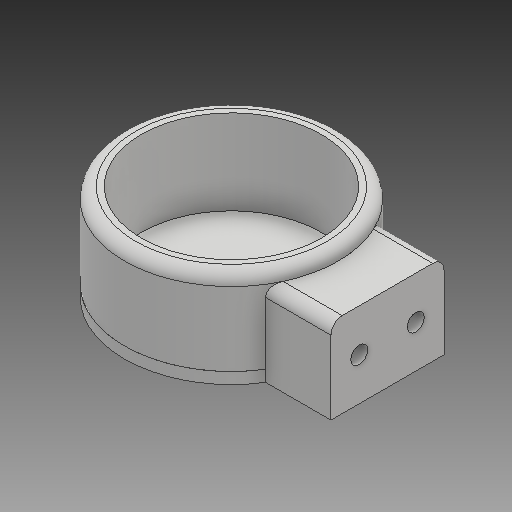
# Autodesk Inventor part: Counter_Support_Ceramic_Base
Saved by Autodesk Inventor 2017 (Build 210142000, 142)
## iProperties
Created: 2020-01-10
Part Number: Counter_Support_Ceramic_Base
Material: Generic
Document SubType Name: Modeling
Designer: Christian
Density: 1 g/cm^3
Appearance: Default
Author: Christian
Autodesk Inventor part; units mm, degrees
ref_plane "YZ Plane" through (0, 0, 0) normal (1, 0, 0) x (0, 1, 0)
ref_plane "XZ Plane" through (0, 0, 0) normal (0, 1, 0) x (-1, 0, 0)
ref_plane "XY Plane" through (0, 0, 0) normal (0, 0, 1) x (1, 0, 0)
sketch "Tube_Base_Skt" plane through (0, 0, 0) normal (0, 0, 1) x (1, 0, 0)
  circle A0 centre (0, 0) radius 18.9
  dimension "d5" = 37.8
  constraints: 1 centre point, 1 coincident
  measures "d5" diameter of A0
extrude "Tube_Base" add sketch "Tube_Base_Skt" along normal blind 2
sketch "Tube_Core_Skt" plane through (0, 0, 2) normal (0, 0, 1) x (1, 0, 0)
  circle A0 centre (0, 0) radius 18.9 projected
  circle A1 centre (0, 0) radius 15.9
  dimension "d8" = 3
  constraints: 1 centre point, 1 concentric
  measures "d8" radial gap between concentric circles of A0 A1
extrude "Tube_Core" add sketch "Tube_Core_Skt" along normal blind 15 separate body
sketch "Block_Skt" plane through (0, 0, 0) normal (0, 0, 1) x (1, 0, 0)
  line L0 (16.0378, -10) -> (27.6, -10)
  line L1 (27.6, 10) -> (16.0378, 10)
  line L2 (27.6, -10) -> (27.6, 10)
  line L3 (18.9, 0) -> (27.6, 0) construction
  arc A0 (18.9, 0) -> (16.0378, 10) centre (0, 0) ccw
  circle A1 centre (0, 0) radius 18.9 projected
  line L4 (0, 0) -> (18.9, 0) construction
  arc A2 (16.0378, -10) -> (18.9, 0) centre (0, 0) ccw
  arc A3 (16.0378, 10) -> (16.0378, -10) centre (0, 0) ccw
  dimension "d12" = 8.7
  dimension "d13" = 20
  constraints: 10 end point, 8 point on circle, 3 centre point, 3 horizontal, 2 concentric, 1 midpoint, 1 parallel, 1 vertical
  measures "d12" distance of L3.start L3.end
  measures "d13" distance of L0.end L1.start
extrude "Block" add sketch "Block_Skt" along normal blind 15 contours A1 A0 L1 L2 L0 bodies 1
sketch "Block_Hole_Skt" plane through (27.6, -10, 0) normal (1, 0, 0) x (0, 0, -1)
  circle A0 centre (-7.5, 5) radius 1.5
  circle A1 centre (-7.5, 15) radius 1.5
  line L0 (0, 10) -> (-15, 10) construction
  line L1 (-15, 0) -> (-15, 20) construction
  line L2 (-7.5, 10) -> (-7.5, 20) construction
  line L3 (0, 20) -> (-15, 20) construction
  line L4 (-7.5, 10) -> (-7.5, 0) construction
  line L5 (0, 0) -> (-15, 0) construction
  point P0 (-7.5, 5)
  dimension "d17" = 3
  constraints: 6 end point, 6 midpoint, 2 centre point, 2 coincident, 1 equal radius
  measures "d17" diameter of A0
extrude "Block_Hole" cut sketch "Block_Hole_Skt" against normal up to surface from surface at 0 round surface about axis through (0, 0, 2) along (0, 0, 1) radius 18.9 far side no bodies 1
fillet "Fillet" radius 2 3 edges at (21.8189, -10, 15) (21.8189, 10, 15) (-18.9, 0, 17)
equation "\"d5\" = tube_diam + 2 * tube_wall_width"
equation "\"d6\" = tube_base_height"
equation "\"d8\" = tube_wall_width"
equation "\"d3\" = tube_wall_height"
equation "\"d12\" = -screw_head_height + screw_length - screw_tolerance"
equation "\"d13\" = block_width"
equation "\"d14\" = block_height"
equation "\"d17\" = screw_body_diam"
equation "\"d18\" = block_height"
equation "\"d16\" = fillet"
equation "\"tube_diam\" = 31.8"
equation "\"tube_tolerance\" = 0.25"
equation "\"tube_wall_width\" = 3"
equation "\"tube_wall_height\" = 15"
equation "\"screw_wall_width\" = 2"
equation "\"screw_body_diam\" = 3"
equation "\"screw_head_diam\" = 8.3"
equation "\"screw_head_height\" = 3"
equation "\"screw_spacing\" = 8"
equation "\"fillet\" = 2"
equation "\"tube_base_height\" = 2"
equation "\"screw_tolerance\" = 1"
equation "\"screw_length\" = 12.7"
equation "\"wood_width\" = 15"
equation "\"block_width\" = 20"
equation "\"block_height\" = 15"
equation "\"screw_head_ang\" = 71.666667deg"
equation "\"screw_head_m\" = 71.666667deg"
body "Solid1"
body "Solid2"
